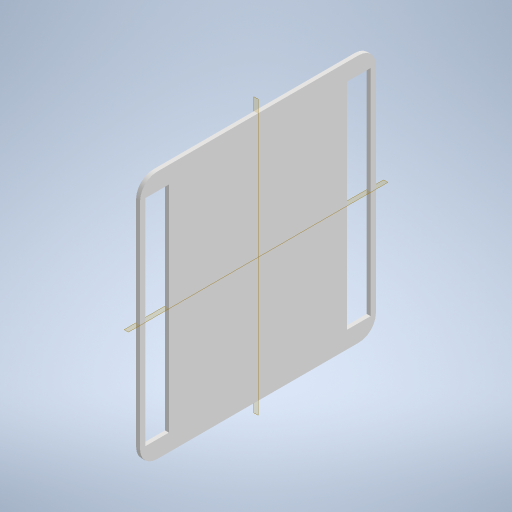
# Autodesk Inventor part: основа_прототип
Saved by Autodesk Inventor 2023 (Build 270158000, 158)
## iProperties
Created: 2025-12-12
Part Number: основа_прототип
Material: Типовые
Document SubType Name: Modeling
Designer: garin
Density: 1 g/cm^3
Appearance: По умолчанию
Author: garin
Autodesk Inventor part; units mm, degrees
ref_plane "YZ Plane" through (0, 0, 0) normal (1, 0, 0) x (0, 1, 0)
sketch "Эскиз1" plane through (0, 0, 0) normal (1, 0, 0) x (0, 1, 0)
  line L0 (95, -77) -> (95, 77)
  line L1 (82, 90) -> (-82, 90)
  line L2 (-95, 77) -> (-95, -77)
  line L3 (-82, -90) -> (82, -90)
  arc A0 (82, -90) -> (95, -77) centre (82, -77) ccw
  arc A1 (-95, -77) -> (-82, -90) centre (-82, -77) ccw
  arc A2 (-82, 90) -> (-95, 77) centre (-82, 77) ccw
  arc A3 (95, 77) -> (82, 90) centre (82, 77) ccw
  line L4 (-82, 90) -> (82, 90)
  line L5 (82, 68) -> (-82, 68)
  line L6 (-82, 68) -> (-82, 86)
  line L7 (-82, 86) -> (82, 86)
  line L8 (-82, -90) -> (82, -90)
  line L9 (82, -86) -> (82, -68)
  line L10 (82, -68) -> (-82, -68)
  line L11 (-82, -68) -> (-82, -86)
  line L12 (-82, -86) -> (82, -86)
  line L13 (82, 86) -> (82, 68)
  line L14 (82, 68) -> (72, 68)
  line L15 (72, 86) -> (82, 86)
  line L16 (-82, 68) -> (-72, 68)
  line L17 (-72, 68) -> (-72, 86)
  line L18 (-72, 86) -> (-82, 86)
  line L19 (-82, 86) -> (-82, 68)
  line L20 (-72, 86) -> (-68.8341, 86)
  line L21 (-68.8341, 86) -> (-68.8341, 84.5)
  line L22 (-68.8341, 84.5) -> (-72, 84.5)
  line L23 (-72, 84.5) -> (-72, 86)
  line L24 (-72, 84.5) -> (-12, 84.5)
  line L25 (-12, 84.5) -> (-12, 69.5)
  line L26 (-12, 69.5) -> (-72, 69.5)
  line L27 (-72, 69.5) -> (-72, 84.5)
  line L28 (82, 86) -> (72, 86)
  line L29 (72, 86) -> (72, 68)
  line L30 (72, 68) -> (82, 68)
  line L31 (82, 68) -> (82, 86)
  line L32 (72, 84.5) -> (12, 84.5)
  line L33 (12, 84.5) -> (12, 69.5)
  line L34 (12, 69.5) -> (72, 69.5)
  line L35 (72, 69.5) -> (72, 84.5)
  line L36 (-42, 68) -> (-54.5, 68)
  line L37 (-54.5, 8) -> (-29.5, 8)
  line L38 (-29.5, 8) -> (-29.5, 68)
  line L39 (-29.5, 68) -> (-54.5, 68)
  line L40 (-54.5, 68) -> (-54.5, 8)
  point P0 (0, 0)
  point P1 (-95, 90)
  point P2 (95, 90)
  point P3 (-95, -90)
  dimension "d6" = 180
  dimension "d7" = 190
  dimension "d8" = 13
  dimension "d9" = 13
  dimension "d11" = 18
  dimension "d19" = 10
  dimension "d20" = 1.5
  dimension "d21" = 60
  dimension "d22" = 15
  dimension "d23" = 10
  dimension "d24" = 60
  dimension "d26" = 60
  dimension "d27" = 25
  constraints: 82 end point, 18 parallel, 13 point on line, 9 perpendicular, 8 point on circle, 8 tangent, 7 horizontal, 4 centre point, 2 equal radius
  measures "d6" distance of point (-95, -90) point (-95, 90)
  measures "d7" distance of point (-95, 90) point (95, 90)
  measures "d8" radius of A0
  measures "d9" radius of A1
  measures "d11" distance of L5.end L6.end
  measures "d19" distance of L18.end L17.end
  measures "d20" distance of L20.end L21.end
  measures "d21" distance of L25.end L26.end
  measures "d22" distance of L24.end L25.end
  measures "d23" distance of L30.end L14.end
  measures "d24" distance of L34.end L33.end
  measures "d26" distance of L37.start L36.end
  measures "d27" distance of L39.end L38.end
extrude "Выдавливание1" add sketch "Эскиз1" along normal blind 3 contours A0 L3 A1 L2 A2 L1 A3 L0 | L38 L37 L40 L5
